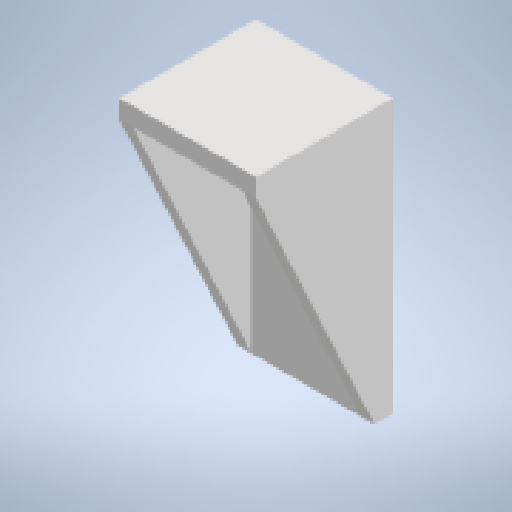
# Autodesk Inventor part: UnionBarras
Saved by Autodesk Inventor 2024 (Build 280153000, 153)
## iProperties
Created: 2023-07-07
Part Number: UnionBarras
Material: Genérico
Document SubType Name: Modeling
Designer: sergi
Density: 1 g/cm^3
Appearance: Valor por defecto
Author: sergi
Autodesk Inventor part; units mm, degrees
ref_plane "YZ Plane" through (0, 0, 0) normal (1, 0, 0) x (0, 1, 0)
ref_plane "XZ Plane" through (0, 0, 0) normal (0, 1, 0) x (-1, 0, 0)
ref_plane "XY Plane" through (0, 0, 0) normal (0, 0, 1) x (1, 0, 0)
sketch "Boceto1" plane through (0, 0, 0) normal (0, 1, 0) x (-1, 0, 0)
  line L0 (-15, -2) -> (15, -2)
  line L1 (15, -2) -> (15, 2)
  line L2 (15, 2) -> (-15, 2)
  line L3 (-15, 2) -> (-15, -2)
  line L4 (-15, -2) -> (15, 2) construction
  line L5 (15, -2) -> (-15, 2) construction
  point P0 (0, 0)
  dimension "d0" = 30
  dimension "d1" = 4
  constraints: 12 end point, 2 midpoint, 2 parallel, 1 horizontal, 1 perpendicular
  measures "d0" distance of L2.end L1.end
  measures "d1" distance of L1.end L0.end
extrude "Extrusión1" add sketch "Boceto1" along normal blind 60
sketch "Boceto2" plane through (-15, 0, 2) normal (0, 0, 1) x (1, 0, 0)
  line L0 (0, 60) -> (30, 60) projected
  line L1 (30, 0) -> (30, 60) projected
  line L2 (0, 60) -> (30, 60)
  line L3 (30, 60) -> (30, 56)
  line L4 (30, 56) -> (0, 56)
  line L5 (0, 56) -> (0, 60)
  point P0 (15, 0)
  dimension "d4" = 4
  constraints: 8 end point, 2 parallel, 1 horizontal, 1 perpendicular, 1 point on line
  measures "d4" distance of L2.end L3.end
extrude "Extrusión2" add sketch "Boceto2" along normal blind 26
sketch "Boceto3" plane through (-15, 0, 2) normal (0, 0, 1) x (1, 0, 0)
  line L0 (0, 0) -> (30, 0) projected
  line L1 (0, 56) -> (30, 56) projected
  line L2 (0, 0) -> (3, 0)
  line L3 (3, 0) -> (3, 56)
  line L4 (3, 56) -> (0, 56)
  line L5 (0, 56) -> (0, 0)
  line L6 (30, 0) -> (27, 0)
  line L7 (27, 0) -> (27, 56)
  line L8 (27, 56) -> (30, 56)
  line L9 (30, 56) -> (30, 0)
  point P0 (15, 0)
  point P1 (3, 0)
  dimension "d7" = 3
  dimension "d8" = 3
  constraints: 16 end point, 4 parallel, 3 point on line, 2 horizontal, 2 perpendicular
  measures "d7" distance of L4.end L3.end
  measures "d8" distance of L7.end L8.end
extrude "Extrusión3" add sketch "Boceto3" along normal blind 26 contours L5 L1 L3 L0 | L7 L1 L9 L0
chamfer "Chaflán1" distance 56 distance2 26 2 edges at (-13.5, 0, 28) (13.5, 0, 28) measured on face at (-14, 38.6667, 28)
sketch "Boceto4" plane through (-12, 56, 2) normal (0, 0, 1) x (1, 0, 0)
  line L0 (27, -56) -> (-3, -56) projected
  line L1 (-3, -56) -> (-3, 4) projected
  line L2 (27, 4) -> (-3, 4) projected
  line L3 (27, -56) -> (27, 4) projected
  line L4 (-3, -56) -> (-3, 4) projected
  line L5 (-3, 4) -> (27, 4)
  line L6 (27, 4) -> (27, -11)
  line L7 (27, -11) -> (-3, -11)
  line L8 (-3, -11) -> (-3, 4)
  line L9 (12, -11) -> (-3, -11)
  line L10 (12, -11) -> (27, -11)
  circle A0 centre (4.5, -11) radius 1.75
  circle A1 centre (19.5, -11) radius 1.75
  line L11 (-3, -56) -> (27, -56)
  line L12 (27, -56) -> (27, -41)
  line L13 (27, -41) -> (-3, -41)
  line L14 (-3, -41) -> (-3, -56)
  line L15 (-3, -41) -> (12, -41)
  line L16 (12, -41) -> (27, -41)
  circle A2 centre (4.5, -41) radius 1.75
  circle A3 centre (19.5, -41) radius 1.75
  point P0 (12, -56)
  dimension "d14" = 30
  dimension "d15" = 15
  dimension "d16" = 3.5
  dimension "d17" = 3.5
  dimension "d18" = 30
  dimension "d19" = 15
  dimension "d20" = 15
  dimension "d21" = 15
  dimension "d22" = 3.5
  dimension "d23" = 3.5
  constraints: 24 end point, 6 midpoint, 4 centre point, 4 parallel, 3 perpendicular, 2 collinear, 2 horizontal
  measures "d14" distance of L6.end L7.end
  measures "d15" distance of L5.end L6.end
  measures "d16" diameter of A0
  measures "d17" diameter of A1
  measures "d18" distance of L13.end L12.end
  measures "d19" distance of L12.end L11.end
  measures "d20" distance of L13.end L15.end
  measures "d21" distance of L15.end L12.end
  measures "d22" diameter of A2
  measures "d23" diameter of A3
hole "Agujero1" at (-7.5, 15, 2) at (7.5, 15, 2) at (7.5, 45, 2) at (-7.5, 45, 2) direction (0, 0, -1) diameter 3.5 end through all countersink diameter 6 countersink angle 90
